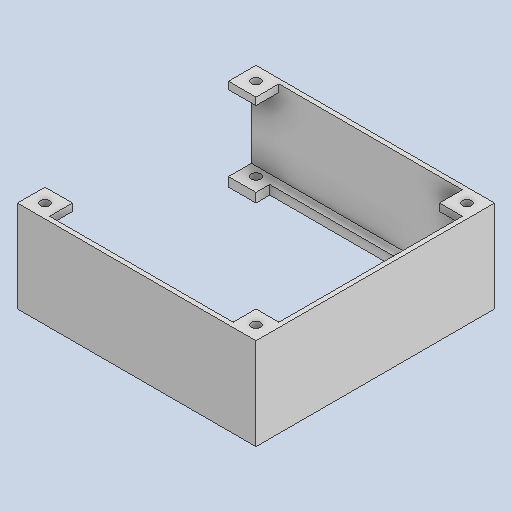
# Autodesk Inventor part: middle
Saved by Autodesk Inventor 2025 (Build 290162000, 162)
## iProperties
Created: 2025-08-07
Part Number: middle
Material: Generic
Document SubType Name: Modeling
Designer: Pravoslav
Density: 1 g/cm^3
Appearance: Default
Author: Pravoslav
Autodesk Inventor part; units mm, degrees
ref_plane "YZ Plane" through (0, 0, 0) normal (1, 0, 0) x (0, 1, 0)
ref_plane "XZ Plane" through (0, 0, 0) normal (0, 1, 0) x (-1, 0, 0)
ref_plane "XY Plane" through (0, 0, 0) normal (0, 0, 1) x (1, 0, 0)
sketch "Sketch1" plane through (0, 0, 0) normal (0, 1, 0) x (-1, 0, 0)
  line L0 (80, 65) -> (-80, 65)
  line L1 (-80, 65) -> (-80, -65)
  line L2 (-80, -65) -> (80, -65)
  line L3 (80, -65) -> (80, 65)
  line L4 (80, 65) -> (-80, -65) construction
  line L5 (-80, 65) -> (80, -65) construction
  line L6 (-72.5, 57.5) -> (42.5, 57.5)
  line L7 (42.5, 57.5) -> (42.5, -57.5)
  line L8 (42.5, -57.5) -> (-72.5, -57.5)
  line L9 (-72.5, -57.5) -> (-72.5, 57.5)
  line L10 (-72.5, 57.5) -> (42.5, -57.5) construction
  line L11 (42.5, 57.5) -> (-72.5, -57.5) construction
  circle A0 centre (42.5, 57.5) radius 2.5
  circle A1 centre (42.5, -57.5) radius 2.5
  circle A2 centre (-72.5, -57.5) radius 2.5
  circle A3 centre (-72.5, 57.5) radius 2.5
  line L12 (50, 65) -> (35, 65)
  line L13 (35, 65) -> (35, 50)
  line L14 (35, 50) -> (50, 50)
  line L15 (50, 50) -> (50, 65)
  line L16 (50, 65) -> (35, 50) construction
  line L17 (35, 65) -> (50, 50) construction
  line L18 (50, -65) -> (35, -65)
  line L19 (35, -65) -> (35, -50)
  line L20 (35, -50) -> (50, -50)
  line L21 (50, -50) -> (50, -65)
  line L22 (50, -65) -> (35, -50) construction
  line L23 (35, -65) -> (50, -50) construction
  line L24 (-80, 65) -> (-65, 65)
  line L25 (-65, 65) -> (-65, 50)
  line L26 (-65, 50) -> (-80, 50)
  line L27 (-80, 50) -> (-80, 65)
  line L28 (-80, 65) -> (-65, 50) construction
  line L29 (-65, 65) -> (-80, 50) construction
  line L30 (-65, -50) -> (-80, -50)
  line L31 (-80, -50) -> (-80, -65)
  line L32 (-80, -65) -> (-65, -65)
  line L33 (-65, -65) -> (-65, -50)
  line L34 (-65, -50) -> (-80, -65) construction
  line L35 (-80, -50) -> (-65, -65) construction
  line L36 (50, 65) -> (50, -65)
  point P0 (0, 0)
  point P1 (-15, 0)
  point P2 (35, 57.5)
  point P3 (35, -57.5)
  point P4 (-65, -57.5)
  point P5 (-72.5, -50)
  point P6 (-72.5, 50)
  point P7 (-65, 57.5)
  dimension "d0" = 160
  dimension "d1" = 130
  dimension "d2" = 115
  dimension "d3" = 115
  dimension "d4" = 7.5
  dimension "d5" = 7.5
  dimension "d6" = 5
  dimension "d7" = 5
  dimension "d8" = 5
  dimension "d9" = 5
  dimension "d12" = 15
  dimension "d13" = 15
  dimension "d14" = 15
  dimension "d15" = 15
  dimension "d16" = 15
  dimension "d17" = 15
  dimension "d18" = 15
  dimension "d19" = 15
  constraints: 74 end point, 12 midpoint, 12 parallel, 6 horizontal, 6 perpendicular, 4 centre point, 4 coincident
  measures "d0" distance of L2.end L1.end
  measures "d1" distance of L1.end L0.end
  measures "d2" distance of L7.end L8.end
  measures "d3" distance of L6.end L7.end
  measures "d4" distance between parallel lines of L1 L9
  measures "d5" distance between parallel lines of L0 L6
  measures "d6" diameter of A0
  measures "d7" diameter of A1
  measures "d8" diameter of A2
  measures "d9" diameter of A3
  measures "d12" distance of L14.end L13.end
  measures "d13" distance of L13.end L12.end
  measures "d14" distance of L19.end L20.end
  measures "d15" distance of L18.end L19.end
  measures "d16" distance of L25.end L26.end
  measures "d17" distance of L24.end L25.end
  measures "d18" distance of L32.end L1.end
  measures "d19" distance of L1.end L30.end
extrude "Extrusion1" add sketch "Sketch1" along normal blind 5 contours L15 L14 L7 A0 L6 L13 L0 | L13 L6 L25 L0 | L2 L19 L8 A1 L7 L20 L21 | L25 L6 A3 L9 L26 L1 L0 | L6 A0 L7 L14 L13 | L2 L33 L8 L19 | L25 L26 L9 A3 L6 | L7 A1 L8 L19 L20 | L2 L1 L30 L9 A2 L8 L33 | L26 L9 L30 L1 | L8 A2 L9 L30 L33
sketch "Sketch2" plane through (0, 5, 0) normal (0, 1, 0) x (1, 0, 0)
  line L0 (80, 65) -> (-50, 65) projected
  line L1 (-50, 65) -> (-50, 50) projected
  line L2 (80, 65) -> (-50, 65)
  line L3 (-50, 65) -> (-50, 62.5)
  line L4 (-50, 62.5) -> (80, 62.5)
  line L5 (80, 62.5) -> (80, 65)
  line L6 (-50, -65) -> (80, -65) projected
  line L7 (80, 65) -> (77.5, 65)
  line L8 (77.5, 65) -> (77.5, -65)
  line L9 (77.5, -65) -> (80, -65)
  line L10 (80, -65) -> (80, 65)
  line L11 (80, -65) -> (-50, -65)
  line L12 (-50, -65) -> (-50, -62.5)
  line L13 (-50, -62.5) -> (80, -62.5)
  line L14 (80, -62.5) -> (80, -65)
  point P0 (0, 0)
  point P1 (80, 62.5)
  point P2 (77.5, 62.5)
  point P3 (77.5, -62.5)
  dimension "d20" = 2.5
  dimension "d21" = 2.5
  dimension "d22" = 2.5
  constraints: 24 end point, 6 parallel, 3 horizontal, 3 perpendicular, 3 point on line
  measures "d20" distance of L3.end L2.end
  measures "d21" distance of L9.end L8.end
  measures "d22" distance of L11.end L12.end
extrude "Extrusion2" add sketch "Sketch2" along normal blind 45
sketch "Sketch3" plane through (0, 50, 0) normal (0, 1, 0) x (1, 0, 0)
  line L0 (80, -65) -> (80, 65) projected
  line L1 (65, 50) -> (72.5, 50) projected
  line L2 (80, 65) -> (65, 65)
  line L3 (65, 65) -> (65, 50)
  line L4 (65, 50) -> (80, 50)
  line L5 (80, 50) -> (80, 65)
  line L6 (72.5, -50) -> (65, -50) projected
  line L7 (-50, -65) -> (80, -65) projected
  line L8 (65, -50) -> (80, -50)
  line L9 (80, -50) -> (80, -65)
  line L10 (80, -65) -> (65, -65)
  line L11 (65, -65) -> (65, -50)
  line L12 (-50, -65) -> (-35, -65)
  line L13 (-35, -65) -> (-35, -50)
  line L14 (-35, -50) -> (-50, -50)
  line L15 (-50, -50) -> (-50, -65)
  line L16 (-50, 62.5) -> (-50, 50) projected
  line L17 (-50, 50) -> (-35, 50)
  line L18 (-35, 50) -> (-35, 65)
  line L19 (-35, 65) -> (-50, 65)
  line L20 (-50, 65) -> (-50, 50)
  circle A0 centre (72.5, 57.5) radius 2.5
  circle A1 centre (72.5, -57.5) radius 2.5 projected
  circle A2 centre (72.5, -57.5) radius 2.5
  circle A3 centre (-42.5, -57.5) radius 2.5 projected
  circle A4 centre (-42.5, -57.5) radius 2.5
  circle A5 centre (-42.5, 57.5) radius 2.5
  point P0 (0, 0)
  dimension "d25" = 15
  dimension "d26" = 15
  dimension "d27" = 5
  dimension "d28" = 5
  dimension "d29" = 5
  dimension "d30" = 5
  constraints: 32 end point, 8 parallel, 4 centre point, 4 horizontal, 4 perpendicular, 4 point on line, 2 coincident
  measures "d25" distance of L14.end L13.end
  measures "d26" distance between parallel lines of L16 L18
  measures "d27" diameter of A0
  measures "d28" diameter of A2
  measures "d29" diameter of A4
  measures "d30" diameter of A5
extrude "Extrusion3" add sketch "Sketch3" against normal blind 4
equation "\"d10\" = d6"
body "Solid1"
